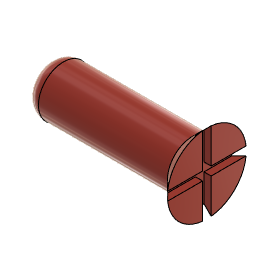
сборка кубсат 2023 v2 (Autodesk Fusion 360 archive; units mm, degrees)
design "болт"
Autodesk Fusion 360 part; units mm, degrees
sketch "Sketch1" plane through (0, 0, 0) normal (1, 0, 0) x (0, 1, 0)
  circle A0 centre (0, 0) radius 1.75
  dimension "d1" = 3.5
  constraint coincident A0.centre origin
  measures "d1" diameter of A0
extrude "Extrude1" add sketch "Sketch1" along normal blind 10
sketch "Sketch2" plane through (10, 0, 0) normal (1, 0, 0) x (0, 1, 0)
  circle A0 centre (0, 0) radius 1.75
  circle A1 centre (0, 0) radius 2.75
  dimension "d4" = 5.5
  constraint concentric A0 A1
  measures "d4" diameter of A1
extrude "Extrude2" add sketch "Sketch2" along normal blind 1 contours A0 | A1
chamfer "Chamfer1" distance 1 angle 45 1 edges at (10, -2.5639, -0.9944)
fillet "Fillet1" radius 1 1 edges at (0, -1.6316, -0.6328)
sketch "Sketch3" plane through (11, 0, 0) normal (1, 0, 0) x (0, 1, 0)
  circle A0 centre (0, 0) radius 2.75
  line L0 (0, 0) -> (0, 4)
  line L1 (0, 4) -> (0, -3.5)
  line L2 (-3, 0) -> (4.1242, 0)
  line L3 (-3, 0) -> (-3, 0.3)
  line L4 (-3, 0.3) -> (3.1636, 0.3)
  line L5 (3.1636, 0.3) -> (3.1636, -0.3)
  line L6 (3.1636, -0.3) -> (-3, -0.3)
  line L7 (-3, -0.3) -> (-3, 0)
  line L8 (0, 3) -> (-0.3, 3)
  line L9 (-0.3, 3) -> (-0.3, -3.1)
  line L10 (-0.3, -3.1) -> (0.3, -3.1)
  line L11 (0.3, -3.1) -> (0.3, 3)
  line L12 (0.3, 3) -> (-0.1, 3)
  dimension "d10" = 0.6
  constraint coincident A0.centre L0.start
  constraint vertical L0
  constraint parallel L0 L1
  constraint perpendicular L1 L2
  constraint perpendicular L2 L3
  constraint perpendicular L3 L4
  constraint perpendicular L4 L5
  constraint perpendicular L5 L6
  constraint coincident L1 L8.start
  constraint perpendicular L0 L8
  constraint perpendicular L8 L9
  constraint perpendicular L9 L10
  constraint perpendicular L10 L11
  constraint coincident L8 L12.end
  constraint perpendicular L0 L12
  measures "d10" distance of L4.end L5.end
extrude "Extrude3" cut sketch "Sketch3" against normal blind 0.5 contours A0 L2 L4 L11 | A0 L2 L6 L11 | L1 L2 L6 L11 | L0 L1 L2 L4 L11 | A0 L0 L1 L4 L11 | A0 L1 L6 L11 | L0 L1 L2 L4 L9 | L1 L2 L6 L9 | A0 L0 L1 L4 L9 | A0 L1 L6 L9 | A0 L2 L6 L9 | A0 L2 L4 L9

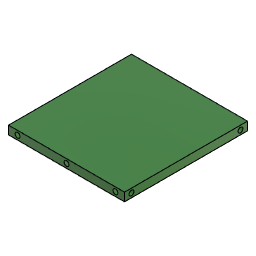
design "боковые"
Autodesk Fusion 360 part; units mm, degrees
sketch "Sketch1" plane through (0, 0, 0) normal (0, 1, 0) x (1, 0, 0)
  line L0 (-45, -25) -> (38, -25)
  line L1 (38, -25) -> (38, -19)
  line L2 (38, -19) -> (-45, -19)
  line L3 (-45, -19) -> (-45, -25)
  dimension "d1" = 83
  dimension "d2" = 6
  constraint horizontal L0
  constraint vertical L1
  constraint horizontal L2
  constraint vertical L3
  measures "d1" distance of L0.start L0.end
  measures "d2" distance of L0.start L2.end
extrude "Extrude1" add sketch "Sketch1" along normal blind 88
sketch "Sketch2" plane through (0, 0, 0) normal (0, -1, 0) x (1, 0, 0)
  line L0 (-45, 25) -> (-45, 19)
  line L1 (-45, 19) -> (38, 19)
  line L2 (38, 19) -> (38, 25)
  line L3 (38, 25) -> (-45, 25)
  line L4 (-3.5, 25) -> (-3.5, 19)
  circle A0 centre (-3.5, 22) radius 1.75
  line L5 (-3.5, 22) -> (-38.5, 22)
  line L6 (-3.5, 22) -> (31.5, 22)
  circle A1 centre (-38.5, 22) radius 1.75
  circle A2 centre (31.5, 22) radius 1.75
  dimension "d5" = 3.5
  dimension "d6" = 35
  dimension "d7" = 35
  dimension "d8" = 3.5
  dimension "d9" = 3.5
  constraint midpoint L3 L4.start
  constraint midpoint L1 L4.end
  constraint midpoint L4 A0.centre
  constraint coincident A0.centre L5.start
  constraint perpendicular L4 L5
  constraint perpendicular L4 L6
  constraint coincident L5.end A1.centre
  constraint coincident L6.end A2.centre
  measures "d5" diameter of A0
  measures "d6" distance of A0.centre L5.end
  measures "d7" distance of A0.centre L6.end
  measures "d8" diameter of A1
  measures "d9" diameter of A2
extrude "Extrude2" cut sketch "Sketch2" against normal blind 132 contours L4 A0 L6 | L4 A0 L5 | L4 A0 L5 | L4 A0 L6 | A1 | A2
sketch "Sketch3" plane through (0, 0, 25) normal (0, 0, 1) x (-1, 0, 0)
  line L0 (45, 0) -> (-38, 0)
  line L1 (-38, 0) -> (-38, -88)
  line L2 (-38, -88) -> (45, -88)
  line L3 (45, -88) -> (45, 0)
sketch "Sketch4" plane through (38, 0, 0) normal (1, 0, 0) x (0, 1, 0)
  line L0 (0, 25) -> (0, 19)
  line L1 (0, 19) -> (88, 19)
  line L2 (88, 19) -> (88, 25)
  line L3 (88, 25) -> (0, 25)
  line L4 (44, 25) -> (44, 22)
  line L5 (44, 22) -> (5, 22)
  circle A0 centre (5, 22) radius 1.75
  circle A1 centre (83, 22) radius 1.75
  dimension "d12" = 3.5
  constraint midpoint L3 L4.start
  constraint perpendicular L3 L4
  constraint perpendicular L0 L5
  constraint coincident L5.end A0.centre
  constraint symmetric L4 A0 A1
  measures "d12" diameter of A0
extrude "Extrude3" cut sketch "Sketch4" against normal blind 127 contours A0 | A1
equation "d3 = 100 mm - 12 mm"

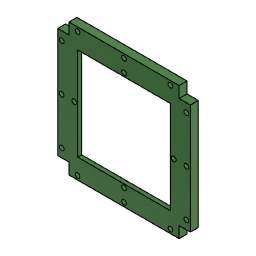
design "2023 кубсат"
Autodesk Fusion 360 part; units mm, degrees
sketch "Sketch1" plane through (0, 0, 0) normal (0, 1, 0) x (1, 0, 0)
  line L0 (-115, -75) -> (-15, -75)
  line L1 (-15, -75) -> (-15, 25)
  line L2 (-15, 25) -> (-115, 25)
  line L3 (-115, 25) -> (-115, -75)
  line L4 (-115, -75) -> (-106.5, -75)
  line L5 (-106.5, -75) -> (-106.5, -66.5)
  line L6 (-106.5, -66.5) -> (-115, -66.5)
  line L7 (-115, -66.5) -> (-115, -75)
  line L8 (-65, -75) -> (-65, -27)
  line L9 (-115, -25) -> (-82, -25)
  line L10 (-106.5, 16.5) -> (-115, 16.5)
  line L11 (-106.5, 25) -> (-106.5, 16.5)
  line L12 (-115, 25) -> (-106.5, 25)
  line L13 (-115, 16.5) -> (-115, 25)
  line L14 (-23.5, -66.5) -> (-15, -66.5)
  line L15 (-15, -66.5) -> (-15, -75)
  line L16 (-15, -75) -> (-115, -75)
  line L17 (-23.5, -75) -> (-23.5, -66.5)
  line L18 (-23.5, 16.5) -> (-15, 16.5)
  line L19 (-23.5, 25) -> (-23.5, 16.5)
  line L20 (-115, 25) -> (-15, 25)
  line L21 (-15, 16.5) -> (-15, 25)
  dimension "d1" = 100
  dimension "d2" = 100
  dimension "d3" = 8.5
  dimension "d4" = 8.5
  constraint horizontal L0
  constraint vertical L1
  constraint horizontal L2
  constraint vertical L3
  constraint horizontal L4
  constraint vertical L5
  constraint horizontal L6
  constraint vertical L7
  constraint midpoint L0 L8.start
  constraint perpendicular L0 L8
  constraint midpoint L3 L9.start
  constraint perpendicular L3 L9
  constraint symmetric L0.start L9 L2.end
  constraint symmetric L4.end L9 L11.start
  constraint symmetric L5.end L9 L10.start
  constraint symmetric L6.end L9 L10.end
  constraint symmetric L0.start L8 L0.end
  constraint symmetric L0.end L8 L0.start
  constraint symmetric L1.end L8 L2.end
  constraint symmetric L2.end L8 L1.end
  constraint symmetric L4.end L8 L17.start
  constraint symmetric L5.end L8 L14.start
  constraint symmetric L6.end L8 L14.end
  constraint symmetric L8 L10.start L18.start
  constraint symmetric L8 L10.end L18.end
  constraint symmetric L8 L11.start L19.start
  constraint symmetric L8 L2.end L1.end
  measures "d1" distance of L0.start L0.end
  measures "d2" distance of L0.start L2.end
  measures "d3" distance of L0.start L4.end
  measures "d4" distance of L0.start L6.end
extrude "Extrude1" add sketch "Sketch1" along normal blind 6 contours L0 L1 L2 L3 L5 L6 L10 L11 L14 L16 L17 L18 L19 L20
sketch "Sketch2" plane through (0, 6, 0) normal (0, 1, 0) x (-1, 0, 0)
  line L0 (23.5, -25) -> (106.5, -25)
  line L1 (106.5, -25) -> (106.5, -16.5)
  line L2 (106.5, -16.5) -> (115, -16.5)
  line L3 (115, -16.5) -> (115, 66.5)
  line L4 (115, 66.5) -> (106.5, 66.5)
  line L5 (106.5, 66.5) -> (106.5, 75)
  line L6 (106.5, 75) -> (23.5, 75)
  line L7 (23.5, 75) -> (23.5, 66.5)
  line L8 (23.5, 66.5) -> (15, 66.5)
  line L9 (15, 66.5) -> (15, -16.5)
  line L10 (15, -16.5) -> (23.5, -16.5)
  line L11 (23.5, -16.5) -> (23.5, -25)
  line L12 (23.5, 75) -> (23.5, 69)
  line L13 (23.5, 72) -> (106.5, 72)
  circle A0 centre (65, 72) radius 1.75
  circle A1 centre (30, 72) radius 1.75
  line L14 (65, 72) -> (65, 73.3681)
  circle A2 centre (100, 72) radius 1.75
  line L15 (65, 75) -> (65, 16.2545)
  line L16 (15, 25) -> (85, 25)
  circle A3 centre (30, -22) radius 1.75
  circle A4 centre (65, -22) radius 1.75
  circle A5 centre (100, -22) radius 1.75
  line L17 (15, -25) -> (39, -1)
  circle A6 centre (18, -10) radius 1.75
  circle A7 centre (18, 25) radius 1.75
  circle A8 centre (18, 60) radius 1.75
  circle A9 centre (112, -10) radius 1.75
  circle A10 centre (112, 25) radius 1.75
  circle A11 centre (112, 60) radius 1.75
  dimension "d7" = 3.5
  dimension "d8" = 3.5
  constraint coincident L6.end L7.start
  constraint coincident L7 L12.end
  constraint perpendicular L6 L12
  constraint midpoint L12 L13.start
  constraint coincident L5 L13.end
  constraint perpendicular L5 L13
  constraint midpoint L13 A0.centre
  constraint coincident L13 A1.centre
  constraint coincident A0.centre L14.start
  constraint perpendicular L13 L14
  constraint symmetric A1 L14 A2
  constraint midpoint L6 L15.start
  constraint perpendicular L13 L15
  constraint midpoint L9 L16.start
  constraint perpendicular L9 L16
  constraint symmetric A0 L16 A4
  constraint symmetric A1 L16 A3
  constraint symmetric A2 L16 A5
  constraint symmetric A3 L17 A6
  constraint symmetric A4 L17 A7
  constraint symmetric A5 L17 A8
  constraint symmetric L15 A6 A9
  constraint symmetric L15 A7 A10
  constraint symmetric L15 A8 A11
  measures "d7" diameter of A0
  measures "d8" diameter of A1
extrude "Extrude2" cut sketch "Sketch2" against normal blind 36 contours L16 A7 | L16 A7 | L13 A2 | L13 A2 | L13 A0 L15 | L13 A0 L15 | L13 A1 | L13 A1 | L13 A0 L14 L15 | L13 A0 L14 L15 | A3 | A4 | A5 | A6 | A8 | A9 | A10 | A11
chamfer "Chamfer1" distance 1 angle 45 12 edges at (-28.3684, 6, 72.6328) (-16.3684, 6, 60.6328) (-16.3684, 6, 25.6328) (-16.3684, 6, -9.3672) (-28.3684, 6, -21.3672) (-63.3684, 6, -21.3672) (-98.3684, 6, -21.3672) (-110.3684, 6, -9.3672) (-110.3684, 6, 25.6328) (-110.3684, 6, 60.6328) (-98.3684, 6, 72.6328) (-63.3684, 6, 72.6328)
sketch "Sketch3" plane through (0, 6, 0) normal (0, 1, 0) x (-1, 0, 0)
  circle A0 centre (100, 72) radius 2.75
  circle A1 centre (112, 25) radius 2.75
  circle A2 centre (100, -22) radius 2.75
  circle A3 centre (30, -22) radius 2.75
  circle A4 centre (18, 25) radius 2.75
  circle A5 centre (30, 72) radius 2.75
  line L0 (23.5, -25) -> (106.5, -25)
  line L1 (106.5, -25) -> (106.5, -16.5)
  line L2 (106.5, -16.5) -> (115, -16.5)
  line L3 (115, -16.5) -> (115, 66.5)
  line L4 (115, 66.5) -> (106.5, 66.5)
  line L5 (106.5, 66.5) -> (106.5, 75)
  line L6 (106.5, 75) -> (23.5, 75)
  line L7 (23.5, 75) -> (23.5, 66.5)
  line L8 (23.5, 66.5) -> (15, 66.5)
  line L9 (15, 66.5) -> (15, -16.5)
  line L10 (15, -16.5) -> (23.5, -16.5)
  line L11 (23.5, -16.5) -> (23.5, -25)
  circle A6 centre (18, 60) radius 2.75
  circle A7 centre (18, -10) radius 2.75
  circle A8 centre (65, -22) radius 2.75
  circle A9 centre (112, -10) radius 2.75
  circle A10 centre (112, 60) radius 2.75
  circle A11 centre (65, 72) radius 2.75
  line L12 (25, 65) -> (105, 65)
  line L13 (105, 65) -> (105, -15)
  line L14 (105, -15) -> (25, -15)
  line L15 (25, -15) -> (25, 65)
  constraint horizontal L12
  constraint vertical L13
  constraint horizontal L14
  constraint vertical L15
extrude "Extrude3" cut sketch "Sketch3" against normal blind 3 contours L12 L13 L14 L15
sketch "Sketch4" plane through (0, 3, 0) normal (0, 1, 0) x (-1, 0, 0)
  line L0 (25, -15) -> (105, -15)
  line L1 (105, -15) -> (105, 65)
  line L2 (105, 65) -> (25, 65)
  line L3 (25, 65) -> (25, -15)
  line L4 (30, 60) -> (100, 60)
  line L5 (100, 60) -> (100, -10)
  line L6 (100, -10) -> (30, -10)
  line L7 (30, -10) -> (30, 60)
  constraint horizontal L4
  constraint vertical L5
  constraint horizontal L6
  constraint vertical L7
extrude "Extrude4" cut sketch "Sketch4" against normal blind 33 contours L4 L5 L6 L7
sketch "Sketch5" plane through (0, 3, 0) normal (0, 1, 0) x (-1, 0, 0)
  line L0 (100, 60) -> (100, -10)
  line L1 (100, -10) -> (30, -10)
  line L2 (30, -10) -> (30, 60)
  line L3 (30, 60) -> (100, 60)
  line L4 (25, -15) -> (105, -15)
  line L5 (105, -15) -> (105, 65)
  line L6 (105, 65) -> (25, 65)
  line L7 (25, 65) -> (25, -15)
  line L8 (25, 65) -> (30, 60)
  line L9 (65, 65) -> (65, 25)
  line L10 (65, 25) -> (25, 25)
  line L11 (25, 25) -> (27.5, 25)
  line L12 (27.5, 25) -> (27.5, 20)
  circle A0 centre (27.5, 25) radius 1.75
  circle A1 centre (102.5, 25) radius 1.75
  circle A2 centre (65, 62.5) radius 1.75
  circle A3 centre (65, -12.5) radius 1.75
  dimension "d16" = 2.5
  dimension "d17" = 3.5
  constraint coincident L6.end L7.start
  constraint coincident L2.end L3.start
  constraint midpoint L6 L9.start
  constraint perpendicular L6 L9
  constraint midpoint L7 L10.end
  constraint perpendicular L7 L10
  constraint perpendicular L7 L11
  constraint perpendicular L10 L12
  constraint coincident L11.end L12.start
  constraint symmetric L9 A0 A1
  constraint symmetric L8 A0 A2
  constraint symmetric L8 A1 A3
  measures "d16" distance of L10.end L11.end
  measures "d17" diameter of A0
extrude "Extrude5" cut sketch "Sketch5" against normal blind 35 contours L9 A2 | L9 A2 | L10 L12 A0 | L10 L11 A0 | L10 L11 L12 A0 | A1 | A3

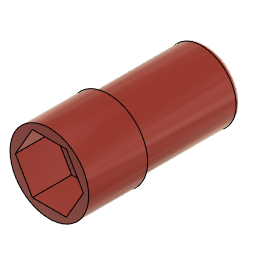
design "под креплениеп полозьев"
Autodesk Fusion 360 part; units mm, degrees
sketch "Sketch1" plane through (0, 0, 0) normal (0, 1, 0) x (1, 0, 0)
  circle A0 centre (0, 0) radius 1.75
  dimension "d1" = 3.5
  constraint coincident A0.centre origin
  measures "d1" diameter of A0
extrude "Extrude1" add sketch "Sketch1" along normal blind 5
sketch "Sketch2" plane through (0, 0, 0) normal (0, -1, 0) x (1, 0, 0)
  circle A0 centre (0, 0) radius 1.75
  circle A1 centre (0, 0) radius 2
  dimension "d4" = 4
  constraint coincident A0.centre A1.centre
  measures "d4" diameter of A1
extrude "Extrude2" add sketch "Sketch2" along normal blind 3 contours A0 | A1
sketch "Sketch3" plane through (0, -3, 0) normal (0, -1, 0) x (1, 0, 0)
  circle A0 centre (0, 0) radius 2
  line L0 (-0.866, 1.5) -> (-1.7321, 0)
  line L1 (-1.7321, 0) -> (-0.866, -1.5)
  line L2 (-0.866, -1.5) -> (0.866, -1.5)
  line L3 (0.866, -1.5) -> (1.7321, 0)
  line L4 (1.7321, 0) -> (0.866, 1.5)
  line L5 (0.866, 1.5) -> (-0.866, 1.5)
  constraint coincident A0.centre origin
extrude "Extrude3" cut sketch "Sketch3" against normal blind 2 contours L0 L1 L2 L3 L4 L5
fillet "Fillet1" radius 0.25 1 edges at (-1.6316, 5, 0.6328)

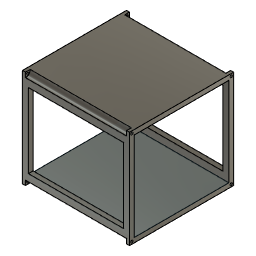
design "картридж поод кубсат"
Autodesk Fusion 360 part; units mm, degrees
sketch "Sketch1" plane through (0, 0, 0) normal (1, 0, 0) x (0, 1, 0)
  line L0 (0, 0) -> (88, 0)
  line L1 (88, 0) -> (88, 83)
  line L2 (88, 83) -> (0, 83)
  line L3 (0, 83) -> (0, 0)
  line L4 (4, 4) -> (84, 4)
  line L5 (84, 4) -> (84, 79)
  line L6 (84, 79) -> (4, 79)
  line L7 (4, 79) -> (4, 4)
  dimension "d1" = 88
  dimension "d2" = 83
  dimension "d3" = -4
  constraint horizontal L0
  constraint vertical L1
  constraint horizontal L2
  constraint vertical L3
  constraint coincident L0.start L3.end
  measures "d1" distance of L0.start L0.end
  measures "d2" distance of L0.start L2.end
extrude "Extrude1" add sketch "Sketch1" along normal blind 2.5
sketch "Sketch2" plane through (2.5, 0, 0) normal (1, 0, 0) x (0, 1, 0)
  line L0 (4, 4) -> (4, 79)
  line L1 (4, 79) -> (84, 79)
  line L2 (84, 79) -> (84, 4)
  line L3 (84, 4) -> (4, 4)
  line L4 (0, 83) -> (0, 0)
  line L5 (0, 0) -> (88, 0)
  line L6 (88, 0) -> (88, 83)
  line L7 (88, 83) -> (0, 83)
  line L8 (0, 83) -> (4, 79)
  circle A0 centre (2, 81) radius 1
  line L9 (44, 83) -> (44, 60)
  line L10 (44, 60) -> (44, 41.5)
  line L11 (44, 41.5) -> (0, 41.5)
  circle A1 centre (86, 81) radius 1
  circle A2 centre (2, 2) radius 1
  circle A3 centre (86, 2) radius 1
  dimension "d6" = 2
  constraint coincident L4.start L7.end
  constraint coincident L0.end L1.start
  constraint midpoint L8 A0.centre
  constraint midpoint L7 L9.start
  constraint perpendicular L1 L9
  constraint parallel L6 L10
  constraint midpoint L4 L11.end
  constraint perpendicular L4 L11
  constraint symmetric A0 L10 A1
  constraint symmetric A0 L11 A2
  constraint symmetric L11 A1 A3
  measures "d6" diameter of A0
extrude "Extrude2" cut sketch "Sketch2" against normal blind 25 contours L8 A0 | L8 A0 | A1 | A2 | A3
sketch "Sketch3" plane through (2.5, 0, 0) normal (1, 0, 0) x (0, 1, 0)
  circle A0 centre (86, 81) radius 1
  circle A1 centre (86, 2) radius 1
  circle A2 centre (2, 81) radius 1
  circle A3 centre (2, 2) radius 1
  line L0 (4, 4) -> (4, 79)
  line L1 (4, 79) -> (84, 79)
  line L2 (84, 79) -> (84, 4)
  line L3 (84, 4) -> (4, 4)
  line L4 (0, 83) -> (0, 0)
  line L5 (0, 0) -> (88, 0)
  line L6 (88, 0) -> (88, 83)
  line L7 (88, 83) -> (0, 83)
  arc A4 (0, 79) -> (4, 83) centre (0.5, 82.5) ccw
  line L8 (44, 83) -> (44, 79)
  line L9 (4, 41.5) -> (0, 41.5)
  arc A5 (84, 83) -> (88, 79) centre (87.5, 82.5) ccw
  arc A6 (4, 0) -> (0, 4) centre (0.5, 0.5) ccw
  arc A7 (88, 4) -> (84, 0) centre (87.5, 0.5) ccw
  constraint coincident L7 A4.end
  constraint coincident L4 A4.start
  constraint midpoint L7 L8.start
  constraint midpoint L1 L8.end
  constraint midpoint L0 L9.start
  constraint midpoint L4 L9.end
  constraint symmetric A4.start L8 A5.end
  constraint symmetric A4.end L8 A5.start
  constraint symmetric A4 L8 A5
  constraint symmetric A4.start L9 A6.end
  constraint symmetric A4.end L9 A6.start
  constraint symmetric A4 L9 A6
  constraint symmetric L9 A5.end A7.start
  constraint symmetric L9 A5.start A7.end
  constraint symmetric L9 A5 A7
extrude "Extrude3" add sketch "Sketch3" along normal blind 85.5 contours L0 L1 L2 L3 L4 L5 L6 L7 L8 L9 A5 A6 A7 | L0 L1 L4 L7 A4 L8 L9
sketch "Sketch4" plane through (88, 0, 0) normal (1, 0, 0) x (0, 1, 0)
  line L0 (84, 79) -> (84, 4)
  line L1 (84, 4) -> (4, 4)
  line L2 (4, 4) -> (4, 79)
  line L3 (4, 79) -> (84, 79)
  line L4 (84, 83) -> (4, 83)
  arc A0 (0, 79) -> (4, 83) centre (0.5, 82.5) ccw
  line L5 (0, 79) -> (0, 4)
  arc A1 (4, 0) -> (0, 4) centre (0.5, 0.5) ccw
  line L6 (4, 0) -> (84, 0)
  arc A2 (88, 4) -> (84, 0) centre (87.5, 0.5) ccw
  line L7 (88, 4) -> (88, 79)
  arc A3 (84, 83) -> (88, 79) centre (87.5, 82.5) ccw
  line L8 (0, 83) -> (88, 83)
  line L9 (88, 83) -> (88, 0)
  line L10 (88, 0) -> (0, 0)
  line L11 (0, 0) -> (0, 83)
  dimension "d11" = 88
  dimension "d12" = 83
  constraint horizontal L8
  constraint vertical L9
  constraint horizontal L10
  constraint vertical L11
  measures "d11" distance of L8.start L8.end
  measures "d12" distance of L8.start L10.end
extrude "Extrude4" add sketch "Sketch4" along normal blind 2.5
sketch "Sketch5" plane through (0, 0, 0) normal (-1, 0, 0) x (0, -1, 0)
  circle A0 centre (-86, 81) radius 1
  circle A1 centre (-86, 2) radius 1
  circle A2 centre (-2, 81) radius 1
  circle A3 centre (-2, 2) radius 1
  line L0 (-4, 79) -> (-4, 4)
  line L1 (-4, 4) -> (-84, 4)
  line L2 (-84, 4) -> (-84, 79)
  line L3 (-84, 79) -> (-4, 79)
  line L4 (0, 0) -> (0, 83)
  line L5 (0, 83) -> (-88, 83)
  line L6 (-88, 83) -> (-88, 0)
  line L7 (-88, 0) -> (0, 0)
  circle A4 centre (-2, 2) radius 1
  circle A5 centre (-86, 2) radius 1
  circle A6 centre (-86, 81) radius 1
  circle A7 centre (-2, 81) radius 1
  constraint concentric A3 A4
  constraint concentric A1 A5
  constraint concentric A0 A6
  constraint concentric A2 A7
extrude "Extrude5" cut sketch "Sketch5" against normal blind 130 contours A0 A6 | A1 A5 | A2 A7 | A3 A4
sketch "Sketch6" plane through (0, 0, 0) normal (0, 1, 0) x (1, 0, 0)
sketch "Sketch7" plane through (0, 0, 0) normal (0, -1, 0) x (1, 0, 0)
  line L0 (0, 83) -> (0, 0)
  line L1 (0, 0) -> (2.5, 0)
  line L2 (2.5, 0) -> (2.5, 4)
  line L3 (2.5, 4) -> (88, 4)
  line L4 (88, 4) -> (88, 0)
  line L5 (88, 0) -> (90.5, 0)
  line L6 (90.5, 0) -> (90.5, 83)
  line L7 (90.5, 83) -> (88, 83)
  line L8 (88, 83) -> (88, 79)
  line L9 (88, 79) -> (2.5, 79)
  line L10 (2.5, 79) -> (2.5, 83)
  line L11 (2.5, 83) -> (0, 83)
  line L12 (90.5, 41.5) -> (0, 41.5)
  line L13 (90.5, 83) -> (45.25, 83)
  line L14 (45.25, 83) -> (45.25, 0)
  line L15 (5, 10) -> (85.5, 10)
  line L16 (85.5, 10) -> (85.5, 73)
  line L17 (85.5, 73) -> (5, 73)
  line L18 (5, 73) -> (5, 10)
  line L19 (5, 10) -> (85.5, 73) construction
  line L20 (85.5, 10) -> (5, 73) construction
  point P0 (45.25, 41.5)
  dimension "d17" = 45.25
  constraint midpoint L6 L12.start
  constraint midpoint L0 L12.end
  constraint coincident L6.end L7.start
  constraint perpendicular L0 L13
  constraint perpendicular L3 L14
  constraint horizontal L15
  constraint perpendicular L15 L16
  constraint parallel L15 L17
  constraint parallel L16 L18
  constraint coincident L19 P0
  constraint coincident L20 P0
  constraint midpoint L12 P0
  measures "d17" distance of L6.end L13.end
extrude "Extrude6" cut sketch "Sketch7" against normal blind 140 contours L12 L14 L17 L18 | L12 L14 L15 L18 | L12 L14 L16 L17 | L12 L14 L15 L16
sketch "Sketch8" plane through (0, 0, 4) normal (0, 0, 1) x (-1, 0, 0)
  line L0 (0, -84) -> (0, -4)
  line L1 (0, -4) -> (-90.5, -4)
  line L2 (-90.5, -4) -> (-90.5, -84)
  line L3 (-90.5, -84) -> (0, -84)
equation "d9 = 88 mm - 2.5 mm"
equation "d17 = ( 90.5 / 2 ) * 1 mm"

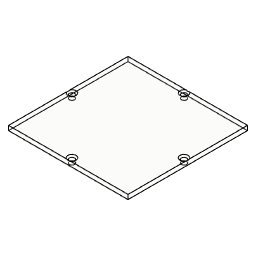
design "стекло"
Autodesk Fusion 360 part; units mm, degrees
sketch "Sketch1" plane through (0, 0, 0) normal (0, 0, 1) x (1, 0, 0)
  line L0 (-65, 60) -> (15, 60)
  line L1 (15, 60) -> (15, -20)
  line L2 (15, -20) -> (-65, -20)
  line L3 (-65, -20) -> (-65, 60)
  dimension "d1" = 80
  dimension "d2" = 80
  constraint horizontal L0
  constraint vertical L1
  constraint horizontal L2
  constraint vertical L3
  measures "d1" distance of L0.start L0.end
  measures "d2" distance of L0.start L2.end
extrude "Extrude1" add sketch "Sketch1" along normal blind 3
sketch "Sketch2" plane through (0, 0, 3) normal (0, 0, 1) x (-1, 0, 0)
  line L0 (65, 20) -> (-15, 20)
  line L1 (-15, 20) -> (-15, -60)
  line L2 (-15, -60) -> (65, -60)
  line L3 (65, -60) -> (65, 20)
  line L4 (62.5, 17.5) -> (-12.5, 17.5)
  line L5 (-12.5, 17.5) -> (-12.5, -57.5)
  line L6 (-12.5, -57.5) -> (62.5, -57.5)
  line L7 (62.5, -57.5) -> (62.5, 17.5)
  line L8 (65, -60) -> (65, -20)
  line L9 (65, -20) -> (25, -20)
  line L10 (25, -20) -> (25, -60)
  line L11 (25, -60) -> (65, -60)
  line L12 (65, -60) -> (65, -20)
  circle A0 centre (62.5, -20) radius 1.75
  circle A1 centre (-12.5, -20) radius 1.75
  line L13 (25, -20) -> (41, -36)
  circle A2 centre (25, -57.5) radius 1.75
  circle A3 centre (25, 17.5) radius 1.75
  dimension "d5" = -2.5
  dimension "d6" = 40
  dimension "d7" = 3.5
  constraint coincident L2.end L3.start
  constraint perpendicular L0 L8
  constraint horizontal L9
  constraint vertical L10
  constraint horizontal L11
  constraint vertical L12
  constraint midpoint L2 L10.end
  constraint midpoint L7 A0.centre
  constraint symmetric L10 A0 A1
  constraint symmetric A0 L13 A2
  constraint symmetric L9 A2 A3
  measures "d6" distance of L2.end L8.end
  measures "d7" diameter of A0
extrude "Extrude2" cut sketch "Sketch2" against normal blind 9 contours L7 L9 A0 | L7 L9 A0 | L7 L9 A0 | L7 L9 A0 | L6 L10 A2 | L6 L10 A2 | L6 L10 A2 | L6 L10 A2 | L4 A3 | L4 A3 | L5 A1 | L5 A1
chamfer "Chamfer1" distance 1 angle 45 4 edges at (-23.3684, -18.1328, 3) (-60.8684, 19.3672, 3) (-23.3684, 56.8672, 3) (14.1316, 19.3672, 3)
